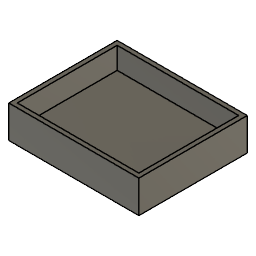
Schalen (Autodesk Fusion 360 design; units mm, degrees)
part number: 2026-01-13-20-48-42-011
Autodesk Fusion 360 part; units mm, degrees
sketch "Skizze1" plane through (0, 0, 0) normal (0, 0, 1) x (1, 0, 0)
  line L0 (0, 0) -> (60, 0)
  line L1 (60, 0) -> (60, 50)
  line L2 (60, 50) -> (0, 50)
  line L3 (0, 50) -> (0, 0)
  dimension "d1" = 60
  dimension "d2" = 50
  constraint horizontal L0
  constraint vertical L1
  constraint horizontal L2
  constraint vertical L3
  constraint coincident L0.start L3.end
  measures "d1" distance of L0.start L0.end
  measures "d2" distance of L0.start L2.end
extrude "Extrusion1" add sketch "Skizze1" along normal blind 5
sketch "Skizze2" plane through (0, 0, 5) normal (0, 0, 1) x (-1, 0, 0)
  line L0 (0, -50) -> (0, 0)
  line L1 (0, 0) -> (-60, 0)
  line L2 (-60, 0) -> (-60, -50)
  line L3 (-60, -50) -> (0, -50)
  line L4 (-58, -2) -> (-58, -48)
  line L5 (-58, -48) -> (-2, -48)
  line L6 (-2, -48) -> (-2, -2)
  line L7 (-2, -2) -> (-58, -2)
  dimension "d5" = -2
extrude "Extrusion2" add sketch "Skizze2" along normal blind 10
scale "Maßstab1" factor 1 about (60, 0, 0) bodies 1
